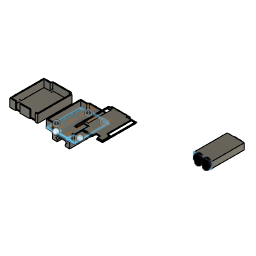
ArduinoOnPicaTinny v1 (Autodesk Fusion 360 design; units mm, degrees)
Autodesk Fusion 360 part; units mm, degrees
sketch "Esquisse1" plane through (0, 0, 0) normal (0, 0, 1) x (1, 0, 0)
  line L0 (-35.3184, -37.4523) -> (17.9616, -37.4523)
  line L1 (17.9616, -37.4523) -> (17.9616, 28.6977)
  line L2 (17.9616, 28.6977) -> (-35.3184, 28.6977) construction
  line L3 (-35.3184, 28.6977) -> (-35.3184, -37.4523)
  line L4 (-20.3184, 31.5477) -> (14.4616, 31.5477)
  line L5 (14.4616, 31.5477) -> (14.4616, -37.4523) construction
  line L6 (14.4616, -37.4523) -> (-22.8684, -37.4523)
  line L7 (-4.2034, 31.5477) -> (-4.2034, -37.4523) construction
  line L8 (17.9616, 40.4753) -> (16.0616, 40.4753) construction
  line L9 (-35.3184, 42.4624) -> (-20.3184, 42.4624) construction
  line L10 (-35.3184, 39.4429) -> (-22.8684, 39.4429) construction
  line L11 (17.9616, 37.2654) -> (14.4616, 37.2654) construction
  line L12 (-20.3184, 42.4624) -> (-20.3184, 28.6977) construction
  line L13 (-20.3184, 28.6977) -> (-20.3184, 31.5477)
  line L14 (16.0616, 40.4753) -> (16.0616, 28.6977) construction
  line L15 (16.0616, 28.6977) -> (14.4616, 31.5477)
  line L16 (-22.8684, 28.6977) -> (-20.3184, 31.5477)
  line L17 (-22.8684, -37.4523) -> (-22.8684, 28.6977) construction
  line L18 (15.6616, -37.4523) -> (15.6616, -25.0523) construction
  circle A0 centre (15.692, -23.7526) radius 1.3
  circle A1 centre (15.692, -23.7526) radius 0.8
  line L19 (16.9616, -24.0323) -> (17.9616, -24.0323) construction
  circle A2 centre (-33.2184, -22.6523) radius 1.3
  circle A3 centre (-33.2184, -22.6523) radius 0.8
  line L20 (-33.2184, -22.6523) -> (-33.2184, -37.4523) construction
  line L21 (-33.2184, -22.6523) -> (-35.3184, -22.6523) construction
  line L22 (-34.5184, -22.6523) -> (-35.3184, -22.6523) construction
  line L23 (-33.2184, -23.9523) -> (-33.2184, -37.4523) construction
  line L24 (-35.3184, 28.6977) -> (-19.3184, 28.6977) construction
  circle A4 centre (-19.3184, 28.6977) radius 1.3
  line L25 (17.9616, 28.6977) -> (11.9616, 28.6977) construction
  circle A5 centre (11.9616, 28.6977) radius 1.3
  circle A6 centre (11.9616, 28.6977) radius 0.8
  circle A7 centre (-19.3184, 28.6977) radius 0.8
  line L26 (17.9616, 28.6977) -> (16.0616, 28.6977) construction
  line L27 (-35.3184, 28.6977) -> (-22.8684, 28.6977)
  line L28 (-25.3184, -31.4523) -> (-16.3184, -31.4523)
  line L29 (-16.3184, -31.4523) -> (-16.3184, -39.4523)
  line L30 (-16.3184, -39.4523) -> (-25.3184, -39.4523)
  line L31 (-25.3184, -39.4523) -> (-25.3184, -31.4523)
  line L32 (14.9616, -25.4523) -> (3.9616, -25.4523)
  line L33 (3.9616, -25.4523) -> (3.9616, -39.4523)
  line L34 (3.9616, -39.4523) -> (14.9616, -39.4523)
  line L35 (14.9616, -39.4523) -> (14.9616, -25.4523)
  line L36 (-35.3184, -31.4523) -> (-25.3184, -31.4523) construction
  line L37 (14.9616, -25.4523) -> (17.9616, -25.4523) construction
  line L38 (-19.9583, -37.4523) -> (-19.9583, -31.4523) construction
  line L39 (5.4938, -37.4523) -> (5.4938, -25.4523) construction
  line L40 (5.573, -37.4523) -> (5.573, -39.4523) construction
  line L41 (-18.5001, -37.4523) -> (-18.5001, -39.4523) construction
  line L42 (16.0616, 28.6977) -> (17.9616, 28.6977)
  line L43 (-21.2126, 33.5477) -> (15.6324, 33.5477)
  line L44 (17.2324, 30.6977) -> (15.6324, 33.5477)
  line L45 (17.2324, 30.6977) -> (19.9616, 30.6977)
  line L46 (19.9616, -39.4523) -> (19.9616, 30.6977)
  line L47 (-37.3184, -39.4523) -> (19.9616, -39.4523)
  line L48 (-37.3184, 30.6977) -> (-37.3184, -39.4523)
  line L49 (-37.3184, 30.6977) -> (-23.7626, 30.6977)
  line L50 (-23.7626, 30.6977) -> (-21.2126, 33.5477)
  dimension "d1" = 53.28
  dimension "d2" = 66.15
  dimension "d3" = 69
  dimension "d5" = 1.9
  dimension "d7" = 15
  dimension "d8" = 12.45
  dimension "d9" = 3.5
  dimension "d10" = 12.4
  dimension "d11" = 2.6
  dimension "d12" = -0.5
  dimension "d13" = 1
  dimension "d14" = 2.6
  dimension "d15" = -0.5
  dimension "d19" = 13.5
  dimension "d20" = 0.8
  dimension "d21" = 16
  dimension "d22" = 2.6
  dimension "d23" = 6
  dimension "d24" = 2.6
  dimension "d25" = -0.5
  dimension "d26" = -0.5
  dimension "d27" = 3
  dimension "d28" = 11
  dimension "d29" = 10
  dimension "d30" = 9
  dimension "d31" = 12
  dimension "d34" = 2
  dimension "d35" = 6
  dimension "d36" = 2
  dimension "d37" = 2
  constraint horizontal L0
  constraint vertical L1
  constraint horizontal L2
  constraint vertical L3
  constraint horizontal L4
  constraint vertical L5
  constraint horizontal L6
  constraint vertical L17
  constraint coincident L0 L5.end
  constraint midpoint L6 L7.end
  constraint coincident L1 L8.start
  constraint perpendicular L1 L8
  constraint coincident L3 L9.start
  constraint perpendicular L3 L9
  constraint coincident L3 L10.start
  constraint coincident L10.end L17
  constraint perpendicular L10 L17
  constraint coincident L1 L11.start
  constraint coincident L5 L11.end
  constraint perpendicular L5 L11
  constraint coincident L2 L12.end
  constraint perpendicular L2 L12
  constraint perpendicular L4 L13
  constraint coincident L2 L14.end
  constraint perpendicular L2 L14
  constraint coincident L2 L16.start
  constraint coincident L4 L7.start
  constraint coincident L0 L18.start
  constraint perpendicular L0 L18
  constraint coincident L18.end A0
  constraint coincident A0 L19.start
  constraint coincident L1 L19.end
  constraint perpendicular L1 L19
  constraint coincident A2.centre A3.centre
  constraint coincident L0 L20.end
  constraint perpendicular L0 L20
  constraint coincident L3 L21.end
  constraint perpendicular L3 L21
  constraint coincident L21 L22.start
  constraint coincident A2 L22.start
  constraint coincident A2 L23.start
  constraint coincident L20 L23.start
  constraint perpendicular L3 L24
  constraint coincident L24.end A4.centre
  constraint perpendicular L1 L25
  constraint coincident L25.end A5.centre
  constraint horizontal L28
  constraint vertical L29
  constraint horizontal L30
  constraint vertical L31
  constraint horizontal L32
  constraint vertical L33
  constraint horizontal L34
  constraint vertical L35
  constraint coincident L3 L36.start
  constraint perpendicular L23 L36
  constraint coincident L1 L37.end
  constraint perpendicular L1 L37
  constraint coincident L6 L38.start
  constraint coincident L28 L38.end
  constraint perpendicular L28 L38
  constraint coincident L6 L39.start
  constraint coincident L32 L39.end
  constraint perpendicular L32 L39
  constraint coincident L0 L40.start
  constraint coincident L34 L40.end
  constraint perpendicular L34 L40
  constraint coincident L0 L41.start
  constraint coincident L30 L41.end
  constraint perpendicular L30 L41
  measures "d1" distance of L0.start L0.end
  measures "d2" distance of L0.start L2.end
  measures "d3" distance of L7.start L7.end
  measures "d5" distance of L8.start L8.end
  measures "d7" distance of L9.start L9.end
  measures "d8" distance of L10.start L10.end
  measures "d9" distance of L11.start L11.end
  measures "d10" distance of L18.start L18.end
  measures "d11" diameter of A0
  measures "d13" distance of L19.start L19.end
  measures "d14" diameter of A2
  measures "d19" distance of L20.end L23.start
  measures "d20" distance of L21.end L22.start
  measures "d21" distance of L2.end L24.end
  measures "d22" diameter of A4
  measures "d23" distance of L1.end L25.end
  measures "d24" diameter of A5
  measures "d27" distance of L32.start L37.end
  measures "d28" distance of L33.end L34.end
  measures "d29" distance of L28.start L36.start
  measures "d30" distance of L28.start L28.end
  measures "d31" distance of L39.start L39.end
  measures "d34" distance of L40.start L40.end
  measures "d35" distance of L38.start L38.end
  measures "d36" distance of L41.start L41.end
extrude "Extrusion2" add sketch "Esquisse1" along normal blind 14 contours L0 L1 L3 L4 L15 L16 L27 L31 L35 L42 L43 L44 L45 L46 L47 L48 L49 L50 | L0 L6 L29 L30 L31 L47 | L0 L6 L29 L33 L47 | L0 L6 L33 L34 L35 L47 makes body 1
extrude "Extrusion1" add sketch "Esquisse1" against normal blind 2 separate body contours L0 L1 L3 L4 L6 L15 L16 L27 L28 L29 L31 L32 L33 L35 L42 | L0 L1 L3 L4 L15 L16 L27 L31 L35 L42 L43 L44 L45 L46 L47 L48 L49 L50 | L0 L6 L28 L29 L31 | L0 L6 L29 L33 L47 | A0 | A1 | A2 | A3 | A4 | A5 | A6 | A7 makes body 2
extrude "Extrusion3" cut sketch "Esquisse1" along normal blind 14 contours L0 L6 L28 L29 L31 | L0 L6 L29 L30 L31 L47 | L0 L6 L32 L33 L35 | L0 L6 L33 L34 L35 L47 bodies 1 makes body 3 at (-9.5584, -39.4523, 4.6667)
extrude "Extrusion4" add sketch "Esquisse1" along normal blind 5 contours A1 | A3 | A6 | A7 bodies 2
extrude "Extrusion5" add sketch "Esquisse1" along normal blind 1 separate body contours L0 L1 L3 L4 L6 L15 L16 L27 L28 L29 L31 L32 L33 L35 L42 makes body 4
move_body "Déplacer1" bodies 4 to x (1, 0, 0) y (0, 1, 0) z (0, 0, 1) at (0, 0, 13)
extrude "Extrusion6" add 3 faces at (-36.6517, 6.6477, 14) (-15.7696, -6.5948, 14) (-9.5584, -38.7856, 14) along direction (0, 0, 1) blind 1 separate body on bodies 1 3 4 makes body 5
combine "Combiner1" operation add target body 4 tool bodies 5
move_body "Déplacer2" bodies 4 to x (1, 0, 0) y (0, 1, 0) z (0, 0, 1) at (0, 0, 15)
move_body "Déplacer3" bodies 4 to x (-1, 0, 0) y (0, 1, 0) z (0, 0, -1) at (39.9232, 0, 60)
extrude "Extrusion7" add 2 faces at (-9.5584, -38.7856, 14) (-36.6517, 6.6477, 14) along direction (0, 0, 1) blind 0.5 on bodies 1 3 bodies 3 1 2
sketch "Esquisse2" plane through (0, 0, 0) normal (0, 1, 0) x (1, 0, 0)
  line L0 (232.235, -61.32) -> (235, -64.32)
  line L1 (232.235, -61.32) -> (235, -58.7716)
  line L2 (250.67, -64.32) -> (235, -64.32)
  line L3 (242.835, -61.32) -> (242.835, -60.32)
  line L4 (242.835, -60.32) -> (249.8865, -60.32)
  line L5 (250.67, -64.32) -> (253.435, -61.32)
  line L6 (235, -64.32) -> (235, -55)
  line L7 (250.67, -55) -> (250.67, -64.32)
  line L8 (235, -55) -> (250.67, -55)
  line L9 (235.7835, -60.32) -> (235.7835, -61.32)
  line L10 (249.8865, -60.32) -> (249.8865, -61.32)
  line L11 (242.835, -60.32) -> (235.7835, -60.32)
  line L12 (242.835, -61.32) -> (232.235, -61.32)
  line L13 (242.835, -64.32) -> (242.835, -61.32)
  line L14 (253.435, -61.32) -> (250.67, -58.7716)
  line L15 (242.835, -61.32) -> (253.435, -61.32)
sketch "Esquisse3" plane through (0, 0, 0) normal (0, 1, 0) x (1, 0, 0)
  line L0 (235, -58.7716) -> (235, -55)
  line L1 (235, -55) -> (250.67, -55)
  line L2 (250.67, -55) -> (250.67, -58.7716)
  line L3 (250.67, -58.7716) -> (253.435, -61.32)
  line L4 (253.435, -61.32) -> (250.67, -64.32)
  line L5 (250.67, -64.32) -> (235, -64.32)
  line L6 (235, -64.32) -> (232.235, -61.32)
  line L7 (232.235, -61.32) -> (235, -58.7716)
  line L8 (235, -55) -> (250.67, -55)
  line L9 (250.67, -55) -> (250.67, -67.5613)
  line L10 (250.67, -67.5613) -> (235, -67.5613)
  line L11 (235, -67.5613) -> (235, -55)
  line L12 (235, -67.5613) -> (225, -67.5613)
  line L13 (225, -67.5613) -> (225, -55)
  line L14 (225, -55) -> (235, -55)
  line L15 (235, -55) -> (235, -67.5613)
  line L16 (250.67, -67.5613) -> (260, -67.5613)
  line L17 (260, -67.5613) -> (260, -55)
  line L18 (260, -55) -> (250.67, -55)
  line L19 (250.67, -55) -> (250.67, -67.5613)
  line L20 (234.7, -54.7) -> (250.97, -54.7)
  line L21 (250.97, -54.7) -> (250.97, -58.6401)
  line L22 (250.97, -58.6401) -> (253.8589, -61.3027)
  line L23 (253.8589, -61.3027) -> (250.8015, -64.62)
  line L24 (250.8015, -64.62) -> (234.8685, -64.62)
  line L25 (234.8685, -64.62) -> (231.8111, -61.3027)
  line L26 (231.8111, -61.3027) -> (234.7, -58.6401)
  line L27 (234.7, -58.6401) -> (234.7, -54.7)
  point P0 (235, -58.7716)
  point P1 (235, -55)
  point P2 (250.67, -55)
  point P3 (250.67, -58.7716)
  point P4 (253.435, -61.32)
  point P5 (250.67, -64.32)
  point P6 (235, -64.32)
  point P7 (232.235, -61.32)
  dimension "d58" = -0.3
  constraint coincident P0 L0.start
  constraint coincident P1 L0.end
  constraint coincident P2 L1.end
  constraint coincident P3 L2.end
  constraint coincident P4 L3.end
  constraint coincident P5 L4.end
  constraint coincident P6 L5.end
  constraint coincident P7 L6.end
  constraint horizontal L8
  constraint vertical L9
  constraint horizontal L10
  constraint vertical L11
  constraint horizontal L12
  constraint vertical L13
  constraint horizontal L14
  constraint vertical L15
  constraint horizontal L16
  constraint vertical L17
  constraint horizontal L18
  constraint vertical L19
extrude "Extrusion8" add sketch "Esquisse3" along normal blind 72 separate body contours L6 L7 L11 L15 | L0 L1 L2 L5 L8 L9 L11 L15 L19 | L3 L4 L9 L19 makes body 6
sketch "Esquisse4" plane through (0, 0, 0) normal (0, 1, 0) x (1, 0, 0)
extrude "Extrusion9" add sketch "Esquisse3" along normal blind 68 separate body contours L0 L6 L7 L11 L14 L15 L24 L25 L26 L27 | L5 L9 L11 L15 L19 L24 | L2 L3 L4 L9 L18 L19 L21 L22 L23 L24 | L11 L12 L13 L14 L15 L24 L25 L26 L27 | L9 L10 L11 L15 L19 L24 | L9 L16 L17 L18 L19 L21 L22 L23 L24 makes body 7
extrude "Extrusion10" cut sketch "Esquisse3" along normal blind 72 contours L0 L6 L7 L11 L14 L15 L24 L25 L26 L27 | L5 L9 L11 L15 L19 L24 | L2 L3 L4 L9 L18 L19 L21 L22 L23 L24 bodies 7
copy_body "Copier/Coller des corps1" bodies 7 makes body 8
move_body "Déplacer4" bodies 8 to x (1, 0, 0) y (0, 1, 0) z (0, 0, 1) at (-256.8484, -39.4523, -69.5613)
move_body "Déplacer5" bodies 8 to x (1, 0, 0) y (0, 1, 0) z (0, 0, 1) at (7, 0, 0)
move_body "Déplacer6" bodies 8 to x (1, 0, 0) y (0, 1, 0) z (0, 0, 1) at (0, 2, 0)
copy_body "Copier/Coller des corps2" bodies 1 2 makes body 9 makes body 10
move_body "Déplacer7" bodies 1 2 3 to x (1, 0, 0) y (0, 1, 0) z (0, 0, 1) at (-75, 0, 0)
extrude "Extrusion14" add 1 faces at (11.2949, -25.4523, -0.6667) along direction (0, -1, 0) blind 14 on bodies 10 bodies 10 9
extrude "Extrusion15" add sketch "Esquisse1" along normal blind 5 separate body contours A7 makes body 11
extrude "Extrusion11" add 1 faces at (-63.7051, -25.4523, -0.6667) along direction (0, -1, 0) blind 12 on bodies 2 bodies 2 8 1 3
extrude "Extrusion12" add 1 faces at (-22.578, -37.4523, -8.2733) along direction (0, -1, 0) blind 2 on bodies 8 bodies 2 8
extrude "Extrusion13" cut sketch "Esquisse1" against normal blind 3 contours L0 L6 L29 L30 L31 L47 | L0 L6 L33 L34 L35 L47 bodies 8 2
sketch "Esquisse5" plane through (0, 0, 32) normal (0, 0, 1) x (-1, 0, 0)
  circle A0 centre (-59.2416, -28.6977) radius 1.3
  circle A1 centre (-24.2312, 23.7526) radius 1.3
  circle A2 centre (-27.9616, -28.6977) radius 1.3
  circle A3 centre (-73.1416, 22.6523) radius 1.3
  line L0 (-75.2416, 37.4523) -> (-75.2416, -28.6977)
  line L1 (-75.2416, -28.6977) -> (-62.7916, -28.6977)
  line L2 (-62.7916, -28.6977) -> (-60.2416, -31.5477)
  line L3 (-60.2416, -31.5477) -> (-25.4616, -31.5477)
  line L4 (-25.4616, -31.5477) -> (-23.8616, -28.6977)
  line L5 (-23.8616, -28.6977) -> (-21.9616, -28.6977)
  line L6 (-21.9616, -28.6977) -> (-21.9616, 37.4523)
  line L7 (-21.9616, 37.4523) -> (-24.9616, 37.4523)
  line L8 (-24.9616, 37.4523) -> (-24.9616, 25.4523)
  line L9 (-24.9616, 25.4523) -> (-35.9616, 25.4523)
  line L10 (-35.9616, 25.4523) -> (-35.9616, 37.4523)
  line L11 (-35.9616, 37.4523) -> (-56.2416, 37.4523)
  line L12 (-56.2416, 37.4523) -> (-56.2416, 31.4523)
  line L13 (-56.2416, 31.4523) -> (-65.2416, 31.4523)
  line L14 (-65.2416, 31.4523) -> (-65.2416, 37.4523)
  line L15 (-65.2416, 37.4523) -> (-75.2416, 37.4523)
  line L16 (-21.9616, -25.5492) -> (-30, -25.5492)
  line L17 (-30, -25.5492) -> (-30, 21)
  line L18 (-30, 21) -> (-21.9616, 21)
  line L19 (-21.9616, 21) -> (-21.9616, -25.5492)
  line L20 (-75.2416, -28.6977) -> (-68, -28.6977)
  line L21 (-68, -28.6977) -> (-68, 21)
  line L22 (-68, 21) -> (-75.2416, 21)
  line L23 (-75.2416, 21) -> (-75.2416, -28.6977)
  constraint horizontal L16
  constraint vertical L17
  constraint horizontal L18
  constraint vertical L19
  constraint coincident L6 L16.start
  constraint horizontal L20
  constraint vertical L21
  constraint horizontal L22
  constraint vertical L23
  constraint coincident L0.end L1.start
extrude "Extrusion16" cut sketch "Esquisse5" against normal blind 3 contours L0 L1 L20 L21 L22 L23 | L6 L16 L17 L18 L19 bodies 4
equation "BordureArduino = 0.3 mm"
